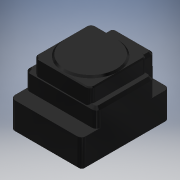
# Autodesk Inventor part: ESC
Saved by Autodesk Inventor 2017.3 (Build 213256000, 256)
## iProperties
Created: 2019-01-11
Part Number: ESC
Material: Generic
Document SubType Name: Modeling
Designer: LSabe
Density: 1 g/cm^3
Appearance: Default
Author: LSabe
Autodesk Inventor part; units mm, degrees
ref_plane "YZ Plane" through (0, 0, 0) normal (1, 0, 0) x (0, 1, 0)
ref_plane "XZ Plane" through (0, 0, 0) normal (0, 1, 0) x (-1, 0, 0)
ref_plane "XY Plane" through (0, 0, 0) normal (0, 0, 1) x (1, 0, 0)
sketch "Sketch1" plane through (0, 0, 0) normal (0, 1, 0) x (-1, 0, 0)
  line L0 (-3.175, 0) -> (-44.323, 0)
  line L1 (-47.498, -3.175) -> (-47.498, -55.245)
  line L2 (-44.323, -58.42) -> (-3.175, -58.42)
  line L3 (0, -55.245) -> (0, -3.175)
  arc A0 (-3.175, -58.42) -> (0, -55.245) centre (-3.175, -55.245) ccw
  arc A1 (-47.498, -55.245) -> (-44.323, -58.42) centre (-44.323, -55.245) ccw
  arc A2 (0, -3.175) -> (-3.175, 0) centre (-3.175, -3.175) ccw
  arc A3 (-44.323, 0) -> (-47.498, -3.175) centre (-44.323, -3.175) ccw
  point P0 (0, 0)
  point P1 (-47.498, -58.42)
  point P2 (-47.498, 0)
  point P3 (0, -58.42)
  dimension "d0" = 47.498
  dimension "d1" = 58.42
  dimension "d2" = 3.175
  dimension "d3" = 3.175
  constraints: 8 end point, 8 point on circle, 8 point on line, 8 tangent, 4 centre point, 2 equal radius, 2 parallel, 1 horizontal, 1 perpendicular
  measures "d0" distance of point (0, -58.42) point (-47.498, -58.42)
  measures "d1" distance of point (-47.498, -58.42) point (-47.498, 0)
  measures "d2" radius of A0
  measures "d3" radius of A2
extrude "Extrusion1" add sketch "Sketch1" along normal blind 19.304
chamfer "Chamfer1" distance 1.651 angle 45 8 edges at (23.749, 0, 0) (46.5681, 0, -0.9299) (47.498, 0, -29.21) (46.5681, 0, -57.4901) (23.749, 0, -58.42) (0.9299, 0, -57.4901) (0, 0, -29.21) (0.9299, 0, -0.9299)
sketch "Sketch3" plane through (0, 19.304, 0) normal (0, 1, 0) x (1, 0, 0)
  line L0 (0, 55.245) -> (0, 3.175) projected
  arc A0 (0, 3.175) -> (3.175, 0) centre (3.175, 3.175) ccw projected
  line L1 (3.175, 0) -> (44.323, 0) projected
  arc A1 (44.323, 0) -> (47.498, 3.175) centre (44.323, 3.175) ccw projected
  line L2 (47.498, 3.175) -> (47.498, 55.245) projected
  arc A2 (47.498, 55.245) -> (44.323, 58.42) centre (44.323, 55.245) ccw projected
  line L3 (44.323, 58.42) -> (3.175, 58.42) projected
  arc A3 (3.175, 58.42) -> (0, 55.245) centre (3.175, 55.245) ccw projected
  line L4 (0, 3.175) -> (0, 55.245) projected
  line L5 (0, 29.21) -> (23.749, 29.21)
  line L6 (0, 29.21) -> (23.749, 29.21) construction
  line L7 (0, 9.779) -> (47.498, 9.779)
  line L8 (47.498, 9.779) -> (47.498, 48.641)
  line L9 (47.498, 48.641) -> (0, 48.641)
  line L10 (0, 48.641) -> (0, 9.779)
  line L11 (0, 9.779) -> (47.498, 48.641) construction
  line L12 (47.498, 9.779) -> (0, 48.641) construction
  point P0 (0, 0)
  dimension "d10" = 38.862
  constraints: 16 end point, 3 midpoint, 2 horizontal, 2 parallel, 1 collinear, 1 perpendicular, 1 point on line
  measures "d10" distance of L8.end L7.end
extrude "Extrusion2" add sketch "Sketch3" along normal blind 12.065 contours L9 L2 L7 L0
fillet "Fillet1" radius 3.175 4 edges at (47.498, 25.3365, -9.779) (0, 25.3365, -9.779) (0, 25.3365, -48.641) (47.498, 25.3365, -48.641)
sketch "Sketch4" plane through (0, 19.304, 0) normal (0, 1, 0) x (1, 0, 0)
  arc A0 (47.498, 45.466) -> (44.323, 48.641) centre (44.323, 45.466) ccw projected
  line L0 (44.323, 48.641) -> (3.175, 48.641) projected
  arc A1 (3.175, 48.641) -> (0, 45.466) centre (3.175, 45.466) ccw projected
  line L1 (0, 45.466) -> (0, 12.954) projected
  arc A2 (0, 12.954) -> (3.175, 9.779) centre (3.175, 12.954) ccw projected
  line L2 (3.175, 9.779) -> (44.323, 9.779) projected
  arc A3 (44.323, 9.779) -> (47.498, 12.954) centre (44.323, 12.954) ccw projected
  line L3 (47.498, 12.954) -> (47.498, 45.466) projected
  line L4 (3.175, 48.641) -> (44.323, 48.641) projected
  arc A4 (47.498, 45.466) -> (44.323, 48.641) centre (44.323, 45.466) ccw projected
  line L5 (47.498, 45.466) -> (47.498, 55.245) projected
  arc A5 (47.498, 55.245) -> (44.323, 58.42) centre (44.323, 55.245) ccw projected
  line L6 (44.323, 58.42) -> (3.175, 58.42) projected
  arc A6 (3.175, 58.42) -> (0, 55.245) centre (3.175, 55.245) ccw projected
  line L7 (0, 55.245) -> (0, 45.466) projected
  arc A7 (3.175, 48.641) -> (0, 45.466) centre (3.175, 45.466) ccw projected
  line L8 (44.323, 48.641) -> (3.175, 48.641) projected
  line L9 (23.749, 48.641) -> (23.749, 58.42)
  line L10 (23.749, 58.42) -> (37.8587, 58.42)
  line L11 (3.175, 58.42) -> (44.323, 58.42) projected
  line L12 (23.749, 58.42) -> (37.8587, 58.42) construction
  line L13 (23.749, 58.42) -> (9.6393, 58.42)
  line L14 (9.6393, 58.42) -> (37.8587, 58.42)
  line L15 (37.8587, 58.42) -> (37.8587, 48.641)
  line L16 (37.8587, 48.641) -> (9.6393, 48.641)
  line L17 (9.6393, 48.641) -> (9.6393, 58.42)
  point P0 (0, 0)
  constraints: 16 end point, 2 collinear, 2 horizontal, 2 midpoint, 2 parallel, 1 perpendicular, 1 point on line, 1 symmetric about line
extrude "Extrusion3" add sketch "Sketch4" along normal blind 16.51 contours L0 L9 L6 L15 | L0 L17 L6 L9
fillet "Fillet2" radius 3.175 2 edges at (9.6393, 27.559, -58.42) (37.8587, 27.559, -58.42)
fillet "Fillet3" radius 3.175 2 edges at (37.8587, 25.3365, -48.641) (9.6393, 25.3365, -48.641)
sketch "Sketch5" plane through (0, 31.369, 0) normal (0, 1, 0) x (1, 0, 0)
  arc A0 (47.498, 45.466) -> (44.323, 48.641) centre (44.323, 45.466) ccw projected
  line L0 (44.323, 48.641) -> (41.0337, 48.641) projected
  arc A1 (37.8587, 51.816) -> (41.0337, 48.641) centre (41.0337, 51.816) ccw projected
  line L1 (37.8587, 48.641) -> (37.8587, 51.816) projected
  line L2 (37.8587, 48.641) -> (9.6393, 48.641) projected
  line L3 (9.6393, 51.816) -> (9.6393, 48.641) projected
  arc A2 (6.4643, 48.641) -> (9.6393, 51.816) centre (6.4643, 51.816) ccw projected
  line L4 (6.4643, 48.641) -> (3.175, 48.641) projected
  arc A3 (3.175, 48.641) -> (0, 45.466) centre (3.175, 45.466) ccw projected
  line L5 (0, 45.466) -> (0, 12.954) projected
  arc A4 (0, 12.954) -> (3.175, 9.779) centre (3.175, 12.954) ccw projected
  line L6 (3.175, 9.779) -> (44.323, 9.779) projected
  arc A5 (44.323, 9.779) -> (47.498, 12.954) centre (44.323, 12.954) ccw projected
  line L7 (47.498, 12.954) -> (47.498, 45.466) projected
  line L8 (0, 45.466) -> (0, 12.954) projected
  line L9 (0, 29.21) -> (24.1894, 29.21)
  line L10 (0, 29.21) -> (24.1894, 29.21) construction
  line L11 (5.3934, 10.16) -> (42.9854, 10.16)
  line L12 (42.9854, 10.16) -> (42.9854, 48.26)
  line L13 (42.9854, 48.26) -> (5.3934, 48.26)
  line L14 (5.3934, 48.26) -> (5.3934, 10.16)
  line L15 (5.3934, 10.16) -> (42.9854, 48.26) construction
  line L16 (42.9854, 10.16) -> (5.3934, 48.26) construction
  point P0 (0, 0)
  dimension "d21" = 37.592
  dimension "d22" = 38.1
  constraints: 16 end point, 3 midpoint, 2 horizontal, 2 parallel, 1 collinear, 1 perpendicular
  measures "d21" distance of L13.end L12.end
  measures "d22" distance of L12.end L11.end
extrude "Extrusion4" add sketch "Sketch5" along normal blind 9.271 contours L14 L13 L12 L11
fillet "Fillet4" radius 3.175 4 edges at (5.3934, 36.0045, -48.26) (5.3934, 36.0045, -10.16) (42.9854, 36.0045, -10.16) (42.9854, 36.0045, -48.26)
sketch "Sketch6" plane through (0, 31.369, 0) normal (0, 1, 0) x (1, 0, 0)
  line L0 (9.6393, 55.245) -> (9.6393, 48.641) projected
  line L1 (37.8587, 48.641) -> (37.8587, 55.245) projected
  line L2 (39.8104, 48.26) -> (8.5684, 48.26) projected
  line L3 (9.6393, 48.641) -> (37.8587, 48.641) projected
  line L4 (37.8587, 48.641) -> (9.6393, 48.641)
  line L5 (9.6393, 48.641) -> (9.6393, 48.26)
  line L6 (9.6393, 48.26) -> (37.8587, 48.26)
  line L7 (37.8587, 48.26) -> (37.8587, 48.641)
  point P0 (0, 0)
  constraints: 8 end point, 2 parallel, 2 point on line, 1 horizontal, 1 perpendicular
extrude "Extrusion5" add sketch "Sketch6" along normal up to surface (4.445 mm away)
chamfer "Chamfer2" distance 1.651 angle 45 16 edges at (9.6393, 35.814, -51.7525) (10.5692, 35.814, -57.4901) (23.749, 35.814, -58.42) (36.9288, 35.814, -57.4901) (37.8587, 35.814, -51.7525) (47.498, 31.369, -29.21) (46.5681, 31.369, -47.7111) (42.6784, 31.369, -48.641) (38.7886, 31.369, -49.5709) (46.5681, 31.369, -10.7089) (23.749, 31.369, -9.779) (0.9299, 31.369, -10.7089) (0, 31.369, -29.21) (0.9299, 31.369, -47.7111) (4.8197, 31.369, -48.641) (8.7094, 31.369, -49.5709)
sketch "Sketch7" plane through (0, 40.64, 0) normal (0, 1, 0) x (1, 0, 0)
  line L0 (7.0444, 13.335) -> (7.0444, 45.085)
  arc A0 (7.0444, 13.335) -> (8.5684, 11.811) centre (8.5684, 13.335) ccw projected
  line L1 (39.8104, 11.811) -> (8.5684, 11.811) projected
  arc A1 (39.8104, 11.811) -> (41.3344, 13.335) centre (39.8104, 13.335) ccw projected
  line L2 (41.3344, 45.085) -> (41.3344, 13.335) projected
  arc A2 (41.3344, 45.085) -> (39.8104, 46.609) centre (39.8104, 45.085) ccw projected
  line L3 (8.5684, 46.609) -> (39.8104, 46.609) projected
  arc A3 (8.5684, 46.609) -> (7.0444, 45.085) centre (8.5684, 45.085) ccw projected
  line L4 (7.0444, 13.335) -> (7.0444, 45.085) projected
  line L5 (7.0444, 29.21) -> (24.1894, 29.21)
  line L6 (7.0444, 29.21) -> (24.1894, 29.21) construction
  circle A4 centre (24.1894, 29.21) radius 18.161
  point P0 (0, 0)
  dimension "d31" = 0
  dimension "d32" = 36.322
  constraints: 6 end point, 5 centre point, 1 coincident, 1 collinear, 1 horizontal, 1 midpoint
  measures "d31" distance between parallel lines of L5 L6
  measures "d32" diameter of A4
extrude "Extrusion6" add sketch "Sketch7" along normal blind 1.0922 contours A4 L0 | L0 A4 L3 L2 L1 | L1 A4 | A4 L3 | L2 A4
chamfer "Chamfer3" distance 1.0922 angle 45 1 edges at (6.0284, 41.7322, -29.21)
chamfer "Chamfer4" distance 0.635 angle 45 8 edges at (24.1894, 40.64, -10.16) (42.0555, 40.64, -11.0899) (42.9854, 40.64, -29.21) (42.0555, 40.64, -47.3301) (24.1894, 40.64, -48.26) (6.3234, 40.64, -47.3301) (5.3934, 40.64, -29.21) (6.3234, 40.64, -11.0899)
fillet "Fillet5" radius 0.254 8 edges at (46.5681, 19.304, -0.9299) (23.749, 19.304, 0) (0.9299, 19.304, -0.9299) (0, 19.304, -8.0645) (47.498, 19.304, -8.0645) (46.5681, 19.304, -57.4901) (39.5034, 19.304, -58.42) (47.498, 19.304, -50.3555)
ref_plane "Midplane" through (23.749, 1.651, -55.245) normal (-1, 0, 0) x (0, 0, 1)
body "Solid1"
